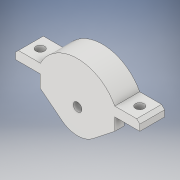
# Autodesk Inventor part: smallWheelStator
Saved by Autodesk Inventor 2019 (Build 230136000, 136)
## iProperties
Created: 2020-12-06
Part Number: smallWheelStator
Material: Пластик АБС
Document SubType Name: Modeling
Designer: Professional
Density: 1.06 g/cm^3
Appearance: Гладкий — белый
Author: Professional
Autodesk Inventor part; units mm, degrees
ref_plane "YZ Plane" through (0, 0, 0) normal (1, 0, 0) x (0, 1, 0)
ref_plane "XZ Plane" through (0, 0, 0) normal (0, 1, 0) x (-1, 0, 0)
ref_plane "XY Plane" through (0, 0, 0) normal (0, 0, 1) x (1, 0, 0)
sketch "Эскиз1" plane through (0, 0, 0) normal (0, 0, 1) x (1, 0, 0)
  circle A0 centre (0, 0) radius 10.75 construction
  line L0 (-40.1576, -0.75) -> (35.328, -0.75) construction
  line L1 (-40.1576, 3.25) -> (35.328, 3.25) construction
  line L2 (-12, 3.25) -> (-20, 3.25)
  line L3 (-20, 3.25) -> (-20, 6.25)
  line L4 (-20, 6.25) -> (0, 6.25)
  line L5 (0, 6.25) -> (0, -8)
  arc A1 (-4.9401, -6.2925) -> (0, -8) centre (0, 0) ccw
  line L6 (12, 3.25) -> (20, 3.25)
  line L7 (20, 3.25) -> (20, 6.25)
  line L8 (20, 6.25) -> (0, 6.25)
  arc A2 (0, -8) -> (4.9401, -6.2925) centre (0, 0) ccw
  line L9 (12, 3.25) -> (12, -0.75)
  line L10 (-12, 3.25) -> (-12, -0.75)
  line L11 (-4.9401, -6.2925) -> (-12, -0.75)
  line L12 (4.9401, -6.2925) -> (12, -0.75)
  dimension "d1" = 21.5
  dimension "d2" = 0.75
  dimension "d3" = 4
  dimension "d4" = 8
  dimension "d5" = 3
  dimension "d6" = 24
  dimension "d7" = 40
  constraints: 26 end point, 5 point on line, 4 point on circle, 4 symmetric about line, 3 centre point, 3 perpendicular, 2 coincident, 2 horizontal, 2 vertical, 1 tangent, 1 other
  measures "d1" diameter of A0
  measures "d2" distance from line of point (0, 0) L0
  measures "d3" distance between parallel lines of L1 L0
  measures "d4" radius of A1
  measures "d5" distance between parallel lines of L1 L4
  measures "d6" diameter of L2.start L5
  measures "d7" diameter of L3 L5
extrude "Выдавливание1" add sketch "Эскиз1" along normal blind 3
sketch "Эскиз2" plane through (0, 0, 0) normal (0, 0, -1) x (-1, 0, 0)
  arc A0 (-4.9401, -6.2925) -> (4.9401, -6.2925) centre (0, 0) ccw projected
  circle A1 centre (0, 0) radius 4
  line L0 (-20, 6.25) -> (20, 6.25) projected
  line L1 (-12, 3.25) -> (-20, 3.25) projected
  line L2 (-20, 3.25) -> (-20, 6.25) projected
  line L3 (-11.5515, 3.25) -> (-20, 3.25)
  line L4 (-20, 3.25) -> (-20, 6.25)
  line L5 (-20, 6.25) -> (-10.2439, 6.25)
  line L6 (10.2439, 6.25) -> (20, 6.25)
  line L7 (20, 6.25) -> (20, 3.25) projected
  line L8 (20, 6.25) -> (20, 3.25)
  line L9 (20, 3.25) -> (11.5515, 3.25)
  arc A2 (-10.2439, 6.25) -> (-11.5515, 3.25) centre (0, 0) ccw
  arc A3 (11.5515, 3.25) -> (10.2439, 6.25) centre (0, 0) ccw
  line L10 (-20, 6.25) -> (20, 6.25) projected
  dimension "d10" = 8
  dimension "d26" = 12
  constraints: 13 end point, 4 point on circle, 3 centre point, 3 coincident, 3 collinear, 2 perpendicular, 2 point on line, 1 concentric, 1 horizontal
  measures "d10" diameter of A1
  measures "d26" radius of A3
extrude "Выдавливание2" add sketch "Эскиз2" along normal blind 2
sketch "Эскиз3" plane through (0, 0, -2) normal (0, 0, -1) x (-1, 0, 0)
  line L0 (-10.2439, 6.25) -> (-20, 6.25) projected
  line L1 (-20, 6.25) -> (-20, 3.25) projected
  line L2 (-20, 3.25) -> (-11.5515, 3.25) projected
  line L3 (11.5515, 3.25) -> (20, 3.25) projected
  line L4 (20, 3.25) -> (20, 6.25) projected
  arc A0 (11.5515, 3.25) -> (10.2439, 6.25) centre (0, 0) ccw projected
  line L5 (20, 6.25) -> (10.2439, 6.25) projected
  arc A1 (-10.2439, 6.25) -> (-11.5515, 3.25) centre (0, 0) ccw projected
extrude "Выдавливание3" add sketch "Эскиз3" along normal blind 3
sketch "Эскиз4" plane through (0, 0, -2) normal (0, 0, -1) x (-1, 0, 0)
  circle A0 centre (0, 0) radius 4 projected
  constraints: 1 coincident
hole "Отверстие1" at (0, 0, -2) direction (0, 0, 1) diameter 2.8 end through all
sketch "Эскиз5" plane through (0, 0, 3) normal (0, 0, 1) x (1, 0, 0)
  arc A0 (10.2439, 6.25) -> (-10.2439, 6.25) centre (0, 0) ccw
  line L0 (20, 6.25) -> (-20, 6.25) projected
  arc A1 (11.9661, 6.25) -> (-11.9661, 6.25) centre (0, 0) ccw
  line L1 (11.9661, 6.25) -> (10.2439, 6.25)
  line L2 (-10.2439, 6.25) -> (-11.9661, 6.25)
  dimension "d22" = 12
  dimension "d23" = 1.5
  constraints: 4 end point, 4 point on circle, 4 point on line, 2 centre point, 2 coincident, 2 collinear
  measures "d22" radius of A0
  measures "d23" radial gap between concentric circles of A1 A0
extrude "Выдавливание4" add sketch "Эскиз5" against normal up to surface (8 mm away) contours A0 L0 A1
sketch "Эскиз6" plane through (0, 0, 3) normal (0, 0, 1) x (1, 0, 0)
  arc A0 (10.2439, 6.25) -> (-10.2439, 6.25) centre (0, 0) ccw projected
  line L0 (10.2439, 6.25) -> (-10.2439, 6.25) projected
extrude "Выдавливание5" add sketch "Эскиз6" against normal up to surface (3 mm away)
sketch "Эскиз7" plane through (20, 6.25, 3) normal (0, 1, 0) x (1, 0, 0)
  line L0 (-40, 8) -> (-40, 0) projected
  line L1 (-31.5515, 8) -> (-8.4485, 8) projected
  line L2 (-20, 8) -> (-20, 0)
  line L3 (-24.9401, 0) -> (-15.0599, 0) projected
  point P0 (-20, 3)
  point P1 (-4, 4)
  point P2 (-36, 4)
  point P3 (-40, 4)
  dimension "d36" = 32
  constraints: 3 midpoint, 2 end point, 2 horizontal alignment, 1 symmetric about line
  measures "d36" distance of point (-36, 4) point (-4, 4)
hole "Отверстие2" at (16, 6.25, -1) at (-16, 6.25, -1) direction (0, -1, 0) diameter 2.8 end through all
chamfer "Фаска1" distance 1 angle 45 2 edges at (20, 6.25, -1) (-20, 6.25, -1)
